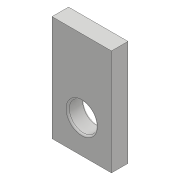
# Autodesk Inventor part: core_case
Saved by Autodesk Inventor 2018 (Build 220112000, 112)
## iProperties
Created: 2018-02-16
Part Number: core_case
Material: Genérico
Document SubType Name: Modeling
Designer: becar
Density: 1 g/cm^3
Appearance: Valor por defecto
Author: becar
Autodesk Inventor part; units mm, degrees
ref_plane "YZ Plane" through (0, 0, 0) normal (1, 0, 0) x (0, 1, 0)
ref_plane "XZ Plane" through (0, 0, 0) normal (0, 1, 0) x (-1, 0, 0)
ref_plane "XY Plane" through (0, 0, 0) normal (0, 0, 1) x (1, 0, 0)
sketch "Boceto1" plane through (0, 0, 0) normal (0, 1, 0) x (-1, 0, 0)
  line L0 (0, 0) -> (18, 0)
  line L1 (18, 0) -> (18, -10)
  line L2 (18, -10) -> (18, -10)
  line L3 (18, -10) -> (18, -22)
  line L4 (18, -22) -> (18, -22)
  line L5 (18, -22) -> (18, -32)
  line L6 (18, -32) -> (0, -32)
  line L7 (0, -32) -> (0, -22)
  line L8 (0, -22) -> (0, -22)
  line L9 (0, -22) -> (0, -10)
  line L10 (0, -10) -> (0, -10)
  line L11 (0, 0) -> (0, -10)
  line L12 (9, -32) -> (9, -22)
  circle A0 centre (9, -22) radius 4.25
  dimension "d0" = 18
  dimension "d1" = 10
  dimension "d2" = 0
  dimension "d3" = 12
  dimension "d4" = 10
  dimension "d5" = 10
  dimension "d6" = 0
  dimension "d10" = 8.5
  constraints: 26 end point, 8 point on line, 7 perpendicular, 1 centre point, 1 coincident, 1 horizontal, 1 midpoint, 1 parallel
  measures "d0" distance of L0.start L0.end
  measures "d1" distance of L0.end L1.end
  measures "d2" distance of L1.end L2.end
  measures "d3" distance of L2.end L3.end
  measures "d4" distance of L4.end L5.end
  measures "d5" distance of L6.end L7.end
  measures "d6" distance of L7.end L8.end
  measures "d10" diameter of A0
extrude "Extrusión2" add sketch "Boceto1" along normal blind 5
fillet "Empalme1" radius 0.5 2 edges at (-4.75, 5, -22) (-4.75, 0, -22)
